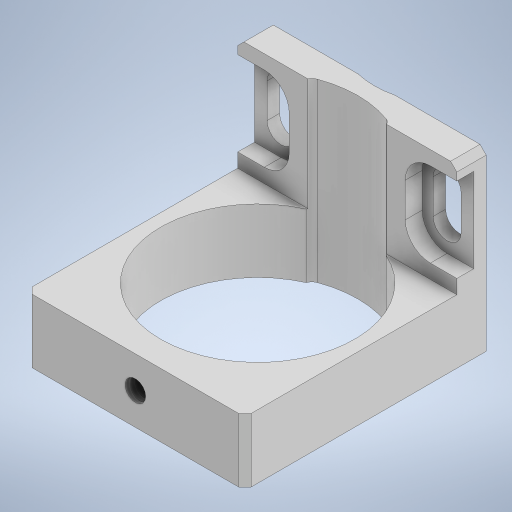
# Autodesk Inventor part: ADAPTER_SM1L03-new
Saved by Autodesk Inventor 2024.2 (Build 282272000, 272)
## iProperties
Created: 2021-02-03
Part Number: ADAPTER_SM1L03-new
Material: Generic
Document SubType Name: Modeling
Designer: maria
Density: 1 g/cm^3
Appearance: Default
Mass: 7.93869 g
Surface Area: 46.2203 cm^2
Volume: 7.93869 cm^3
ItemSpecifications: {"_id":"6021a6fc05ba6b0009d58bc4","finish":"543ef1f380da5b0c476373c1","finish_location":null,"material":"5515e170db035c20ce34af9a","process_initialism":null,"quotes":null,"current_quote":null,"quantity_ordered":10,"features":null,"hardware":null,"threading":null,"part_markings":[],"surface_roughness":null,"tolerance":null,"weld_quantity":null,"Notes":"","certifications":[],"part":null,"revision_num":0,"last_history":null,"inspection_requirement_details":{"inspection_requirement":"std","customer_data_sheet":null},"feedback":null}
Author: maria
Autodesk Inventor part; units mm, degrees
note: some values were not read from the file. Chosen so that the rebuilt part matches the saved one: direction of "Hole4".
ref_plane "YZ Plane" through (0, 0, 0) normal (1, 0, 0) x (0, 1, 0)
ref_plane "XZ Plane" through (0, 0, 0) normal (0, 1, 0) x (-1, 0, 0)
ref_plane "XY Plane" through (0, 0, 0) normal (0, 0, 1) x (1, 0, 0)
sketch "Sketch4" plane through (0, 0, 0) normal (0, 0, 1) x (1, 0, 0)
  line L0 (-17.54, 18) -> (17.54, 18)
  line L1 (17.54, 18) -> (17.54, -10.2)
  line L2 (17.54, -10.2) -> (-17.54, -10.2)
  line L3 (-17.54, -10.2) -> (-17.54, 18)
  point P0 (0, 0)
  dimension "d24" = 28.2
  dimension "WIDTH" = 35.08
  dimension "d26" = 17.54
  dimension "d28" = 10.2
  constraints: 8 end point, 2 parallel, 1 horizontal, 1 perpendicular
  measures "d24" distance of L2.end L0.start
  measures "WIDTH" distance of L1.end L2.end
  measures "d26" distance from line of L3 point (0, 0)
  measures "d28" distance from line of L2 point (0, 0)
extrude "Extrusion3" add sketch "Sketch4" against normal blind 4.7
sketch "Sketch5" plane through (0, 0, 0) normal (0, 0, 1) x (1, 0, 0)
  line L0 (-17.54, -10.2) -> (17.54, -10.2)
  line L1 (17.54, -10.2) -> (17.54, 0)
  line L2 (17.54, 0) -> (-17.54, 0)
  line L3 (-17.54, 0) -> (-17.54, -10.2)
  line L4 (-17.54, 18) -> (-17.54, -10.2) projected
  line L5 (-17.54, -10.2) -> (17.54, -10.2) projected
  line L6 (17.54, -10.2) -> (17.54, 18) projected
  point P0 (0, 0)
  dimension "d31" = 0
  dimension "d32" = 0
  dimension "d33" = 0
  dimension "d34" = 0
  constraints: 8 end point, 2 parallel, 1 horizontal, 1 perpendicular
  measures "d31" distance between parallel lines of L4 L3
  measures "d32" distance between parallel lines of L5 L0
  measures "d33" distance between parallel lines of L6 L1
  measures "d34" distance from line of point (0, 0) L2
extrude "Extrusion4" add sketch "Sketch5" along normal blind 33.93
sketch "Sketch7" plane through (-17.54, -10.2, -4.7) normal (0, -1, 0) x (1, 0, 0)
  circle A0 centre (17.54, 19.05) radius 15.29
  line L0 (35.08, 0) -> (35.08, 38.63) projected
  line L1 (0, 38.63) -> (35.08, 38.63) projected
  line L2 (35.08, 0) -> (0, 0) projected
  line L3 (0, 38.63) -> (0, 0) projected
  circle A1 centre (17.54, 19.05) radius 15.79
  circle A2 centre (12.6611, 5.6453) radius 1.525
  circle A3 centre (22.4189, 5.6453) radius 1.525
  line L4 (17.54, 19.05) -> (17.54, 6.8001)
  line L5 (12.6611, 5.6453) -> (17.54, 19.05)
  line L6 (22.4189, 5.6453) -> (17.54, 19.05)
  point P0 (22.9405, 4.2123)
  point P1 (21.6565, 4.3246)
  point P2 (13.4235, 4.3246)
  point P3 (12.1395, 4.2123)
  point P4 (23.8519, 5.1236)
  point P5 (11.2281, 5.1236)
  dimension "PILOT_HOLE" = 30.58
  dimension "d201" = 19.05
  dimension "d225" = 17.54
  dimension "d226" = 31.58
  dimension "d227" = 20
  dimension "d228" = 20
  dimension "d229" = 3.05
  dimension "d230" = 3.05
  dimension "d231" = 14.265
  dimension "d232" = 14.265
  constraints: 6 end point, 4 centre point, 1 coincident, 1 vertical
  measures "PILOT_HOLE" diameter of A0
  measures "d201" distance from line of L2 A0.centre
  measures "d225" distance from line of L3 A0.centre
  measures "d226" diameter of A1
  measures "d227" angle of L4 L5
  measures "d228" angle of L4 L6
  measures "d229" diameter of A3
  measures "d230" diameter of A2
  measures "d231" distance of L6.start L4.start
  measures "d232" distance of L5.start L4.start
sketch "Sketch9" plane through (0, 0, -4.7) normal (0, 0, -1) x (-1, 0, 0)
  line L0 (17.54, 18) -> (-17.54, 18) projected
  line L1 (17.54, 0) -> (-17.54, 0) projected
  line L2 (0, 5.488) -> (0, 10.988) construction
  line L3 (2.25, 5.488) -> (2.25, 10.988)
  line L4 (-2.25, 10.988) -> (-2.25, 5.488)
  arc A0 (-2.25, 5.488) -> (2.25, 5.488) centre (0, 5.488) ccw
  arc A1 (2.25, 10.988) -> (-2.25, 10.988) centre (0, 10.988) ccw
  line L5 (5.498, 8.238) -> (4.502, 8.238) construction
  line L6 (5.498, 9.288) -> (4.502, 9.288)
  line L7 (4.502, 7.188) -> (5.498, 7.188)
  arc A2 (5.498, 7.188) -> (5.498, 9.288) centre (5.498, 8.238) ccw
  arc A3 (4.502, 9.288) -> (4.502, 7.188) centre (4.502, 8.238) ccw
  point P0 (0, 0)
  point P1 (-5, 8.238)
  point P2 (0, 8.238)
  point P3 (5, 8.238)
  dimension "d183" = 18
  dimension "d185" = 2.25
  dimension "d186" = 5.5
  dimension "d187" = 0
  dimension "d188" = 8.238
  dimension "d189" = 1.05
  dimension "d190" = 0.996
  dimension "d191" = 0
  dimension "d192" = 5
  dimension "d203" = 0
  dimension "d204" = 5
  constraints: 16 end point, 8 point on circle, 8 tangent, 4 centre point, 2 midpoint, 2 parallel, 1 horizontal
  measures "d183" distance between parallel lines of L0 L1
  measures "d185" radius of A1
  measures "d186" distance of L2.start L2.end
  measures "d187" horizontal distance of point (0, 0) point (0, 8.238)
  measures "d188" distance of point (0, 0) point (0, 8.238)
  measures "d189" radius of A3
  measures "d190" distance of L5.start L5.end
  measures "d191" vertical distance of point (0, 8.238) point (5, 8.238)
  measures "d192" distance of point (5, 8.238) point (0, 8.238)
  measures "d203" vertical distance of point (0, 8.238) point (-5, 8.238)
  measures "d204" distance of point (0, 8.238) point (-5, 8.238)
extrude "Extrusion6" cut sketch "Sketch9" against normal blind 2.1 contours A2 L7 A3 L6
extrude "Extrusion7" cut sketch "Sketch7" against normal up to surface (10.2 mm away) contours A0 A3 L6 L5 A2 | A2 A0 | A0 A2 | A3 A0 | A0 A3 | A2 L5 L6 A3 A0 | A0 A3 A1 A2 picked at (17.54, 3.6354)
hole "Hole3" at (5, 8.238, -4.7) direction (0, 0, 1) diameter 2.1 depth 2.1
chamfer "Chamfer10" distance 1 angle 45 4 edges at (17.54, -5.1, 33.93) (-17.54, -5.1, 33.93) (17.54, 18, -2.35) (-17.54, 18, -2.35)
sketch "Sketch13" plane through (-16.54, 18, 0) normal (0, 1, 0) x (1, 0, 0)
  circle A0 centre (16.54, 17.05) radius 12.7
  line L0 (0, 4.7) -> (33.08, 4.7) projected
  point P0 (16.54, 0)
  dimension "d196" = 0
  dimension "d197" = 25.4
  dimension "d224" = 12.35
  constraints: 1 centre point
  measures "d196" horizontal distance of point (16.54, 0) A0.centre
  measures "d197" diameter of A0
  measures "d224" distance from line of L0 A0.centre
extrude "Extrusion11" cut sketch "Sketch13" against normal up to surface (28.2 mm away)
sketch "Sketch14" plane through (0, 0, 33.93) normal (0, 0, 1) x (1, 0, 0)
  line L0 (-17.54, -10.2) -> (17.54, -10.2) projected
  point P0 (0, 0)
  point P1 (0, -5.1)
  point P2 (-16.54, -10.2)
  point P3 (16.54, -10.2)
  dimension "d212" = 0
  dimension "d213" = 5.1
  dimension "d214" = 10.2
  measures "d212" horizontal distance of point (0, 0) point (0, -5.1)
  measures "d213" distance of point (0, 0) point (0, -5.1)
  measures "d214" distance from line of L0 point (0, 0)
hole "Hole4" at (0, -5.1, 33.93) direction (0, 0, -1) diameter 3.302 end up to surface thread size "8-32 UNC" class "2B" standard "ANSI Unified Screw Threads"
sketch "Sketch20" plane through (0, 0, -4.7) normal (0, 0, -1) x (-1, 0, 0)
  line L0 (-17.54, 18) -> (17.54, 18) projected
  line L1 (-17.54, 0) -> (-17.54, 18) projected
  line L2 (-13.29, 6.25) -> (-13.29, 11.75) construction
  line L3 (-11.04, 6.25) -> (-11.04, 11.75)
  line L4 (-15.54, 11.75) -> (-15.54, 6.25)
  arc A0 (-15.54, 6.25) -> (-11.04, 6.25) centre (-13.29, 6.25) ccw
  arc A1 (-11.04, 11.75) -> (-15.54, 11.75) centre (-13.29, 11.75) ccw
  line L5 (5.2784, 0) -> (5.2784, 18) projected
  line L6 (17.54, 18) -> (-17.54, 18) projected
  line L7 (17.54, -10.2) -> (17.54, 18) projected
  line L8 (13.29, 6.25) -> (13.29, 11.75) construction
  line L9 (15.54, 6.25) -> (15.54, 11.75)
  line L10 (11.04, 11.75) -> (11.04, 6.25)
  arc A2 (11.04, 6.25) -> (15.54, 6.25) centre (13.29, 6.25) ccw
  arc A3 (15.54, 11.75) -> (11.04, 11.75) centre (13.29, 11.75) ccw
  circle A4 centre (-5, 8.238) radius 1.05 projected
  point P0 (0, 0)
  point P1 (-13.29, 9)
  point P2 (-5.2784, 18)
  point P3 (17.54, 0)
  point P4 (13.29, 9)
  point P5 (16.54, 18)
  dimension "d251" = 18
  dimension "d252" = 9
  dimension "d253" = 12.2616
  dimension "d254" = 4.25
  dimension "d255" = 4.5
  dimension "d256" = 5.5
  dimension "d257" = 18
  dimension "d258" = 12.2616
  dimension "d259" = 9
  dimension "d261" = 4.5
  dimension "d262" = 5.5
  dimension "d293" = 4.25
  constraints: 16 end point, 8 point on circle, 8 tangent, 4 centre point, 2 midpoint, 2 parallel, 2 vertical
  measures "d251" distance of L1.start L0.start
  measures "d252" distance from line of point (-13.29, 9) L0
  measures "d253" distance of L0.start point (-5.278, 18)
  measures "d254" distance from line of point (-13.29, 9) L1
  measures "d255" diameter of A1
  measures "d256" distance of L2.start L2.end
  measures "d257" distance of L0.end point (17.54, 0)
  measures "d258" distance of L0.end L5.end
  measures "d259" distance from line of L6 point (13.29, 9)
  measures "d261" diameter of A3
  measures "d262" distance of L8.start L8.end
  measures "d293" distance from line of L7 point (13.29, 9)
extrude "Extrusion15" cut sketch "Sketch20" against normal through all contours A0 L4 A1 L3 | A2 L10 A3 L9
sketch "Sketch21" plane through (0, 0, 0) normal (0, 0, 1) x (1, 0, 0)
  line L0 (17.54, 18) -> (-17.54, 18) projected
  line L1 (17.54, 0) -> (17.54, 18) projected
  line L2 (17.54, 0) -> (-17.54, 0) projected
  line L3 (-5.2784, 0) -> (-5.2784, 18) projected
  line L4 (13.29, 11.75) -> (13.29, 6.25) construction
  line L5 (9.29, 11.75) -> (9.29, 6.25)
  line L6 (17.29, 6.25) -> (17.29, 11.75)
  arc A0 (17.29, 11.75) -> (9.29, 11.75) centre (13.29, 11.75) ccw
  arc A1 (9.29, 6.25) -> (17.29, 6.25) centre (13.29, 6.25) ccw
  line L7 (-13.29, 11.75) -> (-13.29, 6.25) construction
  line L8 (-17.29, 11.75) -> (-17.29, 6.25)
  line L9 (-9.29, 6.25) -> (-9.29, 11.75)
  arc A2 (-9.29, 11.75) -> (-17.29, 11.75) centre (-13.29, 11.75) ccw
  arc A3 (-17.29, 6.25) -> (-9.29, 6.25) centre (-13.29, 6.25) ccw
  line L10 (-17.54, 18) -> (-17.54, 0) projected
  line L11 (-13.29, 2.25) -> (-17.54, 2.25)
  line L12 (-13.29, 15.75) -> (-17.54, 15.75)
  line L13 (-17.54, -10.2) -> (-17.54, 18) projected
  line L14 (13.29, 15.75) -> (17.54, 15.75)
  line L15 (13.29, 2.25) -> (17.54, 2.25)
  point P0 (0, 0)
  point P1 (13.29, 9)
  point P2 (5.2784, 18)
  point P3 (-13.29, 9)
  point P4 (-17.54, 15.75)
  point P5 (-16.54, 18)
  dimension "d265" = 9
  dimension "d266" = 4.25
  dimension "d267" = 9
  dimension "d269" = 8
  dimension "d270" = 5.5
  dimension "d271" = 8
  dimension "d272" = 5.5
  dimension "d295" = 4.25
  constraints: 24 end point, 12 point on circle, 9 tangent, 6 point on line, 4 centre point, 3 parallel, 2 midpoint, 2 vertical, 1 horizontal
  measures "d265" distance from line of L0 point (13.29, 9)
  measures "d266" distance from line of L1 point (13.29, 9)
  measures "d267" distance from line of point (-13.29, 9) L2
  measures "d269" diameter of A1
  measures "d270" distance of L4.start L4.end
  measures "d271" diameter of A3
  measures "d272" distance of L7.start L7.end
  measures "d295" distance from line of L10 point (-13.29, 9)
extrude "Extrusion16" cut sketch "Sketch21" against normal blind 2.7 contours L1 L15 A1 L6 A0 L14 | A0 L6 A1 L5 | L12 A2 L8 A3 L11 L10 | A2 L9 A3 L8
sketch "Sketch26" plane through (-17.54, -10.2, -4.7) normal (0, -1, 0) x (1, 0, 0)
  circle A0 centre (17.54, 19.05) radius 15.54
  line L0 (34.4, 0) -> (34.4, 38.38)
  line L1 (0, 38.38) -> (34.4, 38.38)
  line L2 (34.4, 0) -> (0, 0)
  line L3 (0, 0) -> (0, 38.38)
  circle A1 centre (17.54, 19.05) radius 16.04
  circle A2 centre (12.5756, 5.4104) radius 1.525
  circle A3 centre (22.5044, 5.4104) radius 1.525
  line L4 (17.54, 19.05) -> (17.54, 6.8001)
  line L5 (12.5756, 5.4104) -> (17.54, 19.05)
  line L6 (22.5044, 5.4104) -> (17.54, 19.05)
  point P0 (17.54, 4.7)
  point P1 (22.6005, 4.2123)
  point P2 (21.3165, 4.3246)
  point P3 (13.0835, 4.3246)
  point P4 (11.7995, 4.2123)
  point P5 (23.5119, 5.1236)
  point P6 (10.8881, 5.1236)
  point P7 (11.1429, 4.8878)
  point P8 (12.054, 3.9773)
  point P9 (23.026, 3.9773)
  point P10 (23.9371, 4.8878)
  dimension "d314" = 31.08
  dimension "d315" = 19.05
  dimension "d316" = 17.54
  dimension "d317" = 32.08
  dimension "d318" = 20
  dimension "d319" = 20
  dimension "d320" = 3.05
  dimension "d321" = 3.05
  dimension "d322" = 14.515
  dimension "d323" = 14.515
  constraints: 14 end point, 4 centre point, 1 coincident, 1 vertical
  measures "d314" diameter of A0
  measures "d315" distance from line of L2 A0.centre
  measures "d316" distance from line of L3 A0.centre
  measures "d317" diameter of A1
  measures "d318" angle of L4 L5
  measures "d319" angle of L4 L6
  measures "d320" diameter of A3
  measures "d321" diameter of A2
  measures "d322" distance of L6.start L4.start
  measures "d323" distance of L5.start L4.start
extrude "Extrusion19" cut sketch "Sketch26" against normal through all contours A0 A3 L6 L5 A2 | A2 A0 | A0 A2 | A3 A0 | A0 A3 | A2 L5 L6 A3 A0 | A0 A3 A1 A2 picked at (17.54, 3.3865)
equation "\"TOLERANCE\" = 0.05"
equation "\"BEAM_HEIGHT\" = 19.05"
equation "\"d309\" = 19.05"
equation "\"d311\" = 0.05"
equation "\"d324\" = 19.05"
equation "\"d326\" = 0.05"
body "Solid2"
